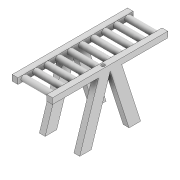
# Autodesk Inventor part: 빨랫대
Saved by Autodesk Inventor 2020 (Build 240168000, 168)
## iProperties
Created: 2022-08-24
Part Number: 빨랫대
Material: 일반
Document SubType Name: Modeling
Designer: 박연호
Density: 1 g/cm^3
Appearance: 기본값
Author: 박연호
Autodesk Inventor part; units mm, degrees
ref_plane "XZ Plane" through (0, 0, 0) normal (0, 1, 0) x (-1, 0, 0)
sketch "스케치1" plane through (0, 0, 0) normal (0, 1, 0) x (-1, 0, 0)
  point P0 (0, 0)
sketch "스케치2" plane through (0, 0, 0) normal (1, 0, 0) x (0, 1, 0)
  line L0 (0, 0) -> (10, 0)
  line L1 (10, 0) -> (10, 100)
  line L2 (10, 100) -> (0, 100)
  line L3 (0, 100) -> (0, 0)
  dimension "d0" = 10
  dimension "d1" = 100
  constraints: 8 end point, 2 parallel, 1 horizontal, 1 perpendicular
  measures "d0" distance of L1.end L2.end
  measures "d1" distance of L0.end L1.end
extrude "돌출1" add sketch "스케치2" along normal blind 10
sketch "스케치3" plane through (0, 0, 0) normal (-1, 0, 0) x (0, 0, 1)
  circle A0 centre (10, 5) radius 5
  line L0 (0, 10) -> (100, 10) projected
  line L1 (0, 0) -> (0, 10) projected
  circle A1 centre (30, 5) radius 5
  circle A2 centre (50, 5) radius 5
  circle A3 centre (70, 5) radius 5
  circle A4 centre (90, 5) radius 5
  dimension "d4" = 10
  dimension "d5" = 5
  dimension "d6" = 10
  dimension "d9" = 20
  constraints: 5 centre point, 1 horizontal, 8 other
  measures "d4" diameter of A0
  measures "d5" distance from line of A0.centre L0
  measures "d6" distance from line of A0.centre L1
  measures "d9" distance of A0.centre A1.centre
extrude "돌출2" add sketch "스케치3" along normal blind 50
sketch "스케치4" plane through (-50, 5, 50) normal (-1, 0, 0) x (0, 0, 1)
  line L0 (-50, -5) -> (-50, 5) projected
  line L1 (50, -5) -> (-50, -5) projected
  line L2 (-50, 5) -> (50, 5)
  line L3 (50, 5) -> (50, -5)
  line L4 (50, -5) -> (-50, -5)
  line L5 (-50, -5) -> (-50, 5)
  constraints: 8 end point, 2 parallel, 1 horizontal, 1 perpendicular
extrude "돌출3" add sketch "스케치4" along normal blind 10
mirror "미러1" about plane through (0, 0, 0) normal (0, 0, -1) of "돌출1", "돌출2", "돌출3"
sketch "스케치5" plane through (-60, 5, 50) normal (-1, 0, 0) x (0, 0, 1)
  line L0 (-50, -5) -> (-30, -5)
  line L1 (50, -5) -> (-150, -5) projected
  line L2 (-30, -5) -> (2.8652, -106.6282)
  line L3 (2.8652, -106.6282) -> (-17.1348, -106.6282)
  line L4 (-17.1348, -106.6282) -> (-50, -5)
  line L5 (-70, -5) -> (-102.8652, -106.6282)
  line L6 (-102.8652, -106.6282) -> (-82.8652, -106.6282)
  line L7 (-82.8652, -106.6282) -> (-50, -5)
  line L8 (-50, -5) -> (-70, -5)
  line L9 (-80, -5) -> (-60, -5) projected
  dimension "d18" = 20
  dimension "d19" = 20
  constraints: 16 end point, 2 equal length, 1 point on line
  measures "d18" distance of L0.start L0.end
  measures "d19" distance of L2.end L3.end
extrude "돌출4" add sketch "스케치5" against normal blind 10
ref_plane "작업 평면3" through (-25, 0, 0) normal (1, 0, 0) x (0, 1, 0)
mirror "미러2" about plane through (-25, 0, 0) normal (1, 0, 0) of "돌출4"
ref_plane "작업 평면4" through (5, 0, 0) normal (1, 0, 0) x (0, 0, -1)
sketch "스케치6" plane through (5, 0, 0) normal (1, 0, 0) x (0, 0, -1)
  line L0 (-32.8652, -101.6282) -> (0, 0) projected
  line L1 (-20, 0) -> (-52.8652, -101.6282) projected
  line L2 (-43.375, -101.6282) -> (-7.276, 10)
  line L3 (-52.8652, -101.6282) -> (-32.8652, -101.6282) projected
  line L4 (-32.8652, -101.6282) -> (-52.8652, -101.6282)
  line L5 (-40.5175, -102.5417) -> (-4.1231, 10)
  line L6 (-10, 10) -> (-30, 10) projected
  line L7 (-10, 10) -> (10, 10) projected
  line L8 (-40.5175, -102.5417) -> (-46.8616, -122.1595)
  line L9 (-43.375, -101.6282) -> (-50.3591, -123.2247)
  line L10 (-46.8616, -122.1595) -> (-50.0146, -122.1595)
  dimension "d25" = 10
  dimension "d26" = 3
  constraints: 12 end point, 4 point on line, 3 collinear, 3 parallel
  measures "d25" distance between parallel lines of L0 L2
  measures "d26" distance between parallel lines of L2 L5
revolve "회전1" cut sketch "스케치6" angle 360 about axis through (5, -101.6282, 43.375) along (0, 0.9514844, -0.307697)
sketch "스케치7" plane through (10, -101.6282, 32.8652) normal (0, -0.307697, -0.9514844) x (-1, 0, 0)
  circle A0 centre (5, 8.9084) radius 4.5
  point P0 (10, 106.8101)
  dimension "d28" = 9
  constraints: 1 centre point
  measures "d28" diameter of A0
extrude "돌출5" cut sketch "스케치7" against normal blind 18
sketch "스케치8" plane through (5, 0, 0) normal (1, 0, 0) x (0, 0, -1)
  point P0 (0, 0)
